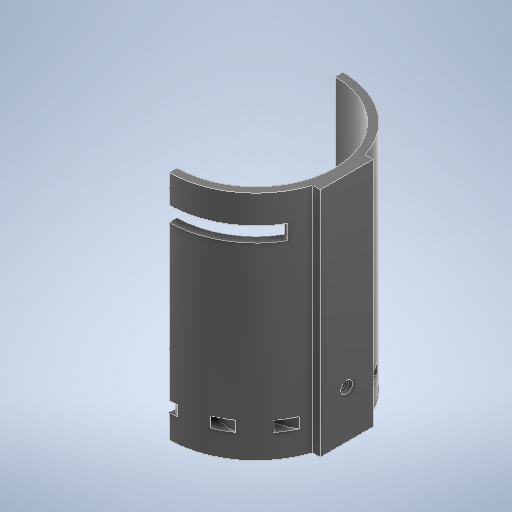
# Autodesk Inventor part: casing_cylindrical
Saved by Autodesk Inventor 2025 (Build 290162000, 162)
## iProperties
Created: 2026-08-03
Part Number: casing_cylindrical
Material: Ogólny
Document SubType Name: Modeling
Designer: zzapa
Density: 1 g/cm^3
Appearance: Gładki — czarny
Author: zzapa
Autodesk Inventor part; units mm, degrees
ref_plane "YZ Plane" through (0, 0, 0) normal (1, 0, 0) x (0, 1, 0)
ref_plane "XZ Plane" through (0, 0, 0) normal (0, 1, 0) x (-1, 0, 0)
sketch "Szkic1" plane through (0, 0, 0) normal (0, 0, 1) x (1, 0, 0)
  line L0 (-6.6, 0) -> (39.6, 0) projected
  line L1 (33, 80) -> (30, 80)
  line L2 (30, 80) -> (30, 0)
  line L3 (30, 0) -> (33, 0)
  line L4 (33, 0) -> (33, 80)
  line L5 (0, -29.6) -> (0, 121.6) projected
  line L6 (33, -8) -> (14, -8)
  line L7 (14, -8) -> (14, 0)
  line L8 (14, 0) -> (33, 0)
  line L9 (33, 0) -> (33, -8)
  line L10 (23, 6) -> (30, 6)
  line L11 (30, 6) -> (30, 0)
  line L12 (30, 0) -> (23, 0)
  line L13 (23, 0) -> (23, 6)
  point P0 (0, 0)
  point P1 (30, 0)
  point P2 (33, 0)
  point P3 (14, 0)
  point P4 (23, 0)
  dimension "d0" = 30
  dimension "d1" = 3
  dimension "d2" = 80
  dimension "d4" = 8
  dimension "d5" = 14
  dimension "d6" = 23
  dimension "d7" = 6
  constraints: 24 end point, 6 parallel, 5 collinear, 3 horizontal, 3 perpendicular
  measures "d0" distance from line of point (0, 0) L2
  measures "d1" distance of L1.start L1.end
  measures "d2" distance of L3.end L1.start
  measures "d4" distance of L6.end L7.end
  measures "d5" distance between parallel lines of L5 L7
  measures "d6" distance between parallel lines of L5 L13
  measures "d7" distance of L12.end L10.start
revolve "Obrót1" add sketch "Szkic1" angle 360 about axis through (0, -10, 0) along (0, 1, 0)
sketch "Szkic2" plane through (0, -8, 0) normal (0, -1, 0) x (1, 0, 0)
  circle A0 centre (0, 0) radius 33 projected
  line L0 (-34.4484, 10) -> (-31.4484, 10)
  line L1 (-31.4484, 10) -> (-31.4484, -10)
  line L2 (-31.4484, -10) -> (-34.4484, -10)
  line L3 (-34.4484, -10) -> (-34.4484, 10)
  line L4 (0, -46.2) -> (0, 46.2) projected
  line L5 (34.4484, 10) -> (31.4484, 10)
  line L6 (31.4484, 10) -> (31.4484, -10)
  line L7 (31.4484, -10) -> (34.4484, -10)
  line L8 (34.4484, -10) -> (34.4484, 10)
  line L9 (-49.8666, 0) -> (49.8666, 0) projected
  point P0 (-31.4484, 0)
  dimension "d10" = 20
  dimension "d11" = 3
  constraints: 16 end point, 4 symmetric about line, 2 parallel, 1 horizontal, 1 midpoint, 1 perpendicular, 1 point on line, 2 other
  measures "d10" distance of L2.end L0.start
  measures "d11" distance from line of L3 point (-31.448, 0)
extrude "Wyciągnięcie proste1" add sketch "Szkic2" against normal up to surface (88 mm away) contours L9 L6 A0 | L9 L8 L7 A0 | A0 L6 L9 | A0 L5 L8 L9 | L1 L9 A0 | A0 L9 L3 L0 | L2 L3 L9 A0 | A0 L9 L1
ref_plane "Płaszczyzna konstrukcyjna1" through (0, 36, 33) normal (0, 0, 1) x (1, 0, 0)
sketch "Szkic3" plane through (0, 36, 33) normal (0, 0, 1) x (1, 0, 0)
  line L0 (3.5, -35) -> (-3.5, -35)
  line L1 (-3.5, -35) -> (-3.5, -31)
  line L2 (-3.5, -31) -> (3.5, -31)
  line L3 (3.5, -31) -> (3.5, -35)
  line L4 (23, -36) -> (-23, -36) projected
  line L5 (23, -30) -> (-23, -30) projected
  line L6 (0, -30) -> (0, -36)
  line L7 (-3.5, -31) -> (3.5, -35)
  point P0 (0, -35)
  point P1 (0, -33)
  dimension "d17" = 4
  dimension "d18" = 7
  constraints: 12 end point, 4 midpoint, 2 parallel, 1 horizontal, 1 perpendicular
  measures "d17" distance of L2.end L0.start
  measures "d18" distance of L1.end L2.end
sketch "Szkic4" plane through (0, 6, 0) normal (0, 1, 0) x (1, 0, 0)
  arc A0 (-31.4484, -10) -> (31.4484, -10) centre (0, 0) ccw projected
  arc A1 (0, 0) -> (0, -33) centre (11.3027, -16.5) ccw
  dimension "d19" = 20
  constraints: 4 point on circle, 1 centre point, 1 coincident
  measures "d19" radius of A1
sweep "Przeciągnięcie1" cut profiles "Szkic3" path "Szkic4" path curves A1
pattern_circular "Szyk kołowy1" count 12 over 360 about axis through (0, -10, 0) along (0, 1, 0) of "Przeciągnięcie1" skipped copies 4 10
sketch "Szkic5" plane through (-34.4484, -8, 10) normal (0, -1, 0) x (1, 0, 0)
  line L0 (34.4484, -56.2) -> (34.4484, 36.2) projected
  point P0 (34.4484, -10)
  point P1 (34.4484, 9)
  point P2 (17.9939, -19.5)
  point P3 (50.9029, -19.5)
  dimension "d20" = 19
  dimension "d23" = 360
  constraints: 1 point on line, 4 other
  measures "d20" distance of point (34.448, -10) point (34.448, 9)
hole "Otwór1" at (0, -8, 19) at (-16.4545, -8, -9.5) at (16.4545, -8, -9.5) direction (0, 1, 0) diameter 2.9 end through all
sketch "Szkic6" plane through (-34.4484, -8, -10) normal (-1, 0, 0) x (0, 0, 1)
  line L0 (10, -17.6) -> (10, 105.6) projected
  line L1 (20, 0) -> (0, 0) projected
  point P0 (10, 8)
  point P1 (10, 18.1)
  dimension "d35" = 18.1
  constraints: 1 point on line
  measures "d35" distance from line of L1 point (10, 18.1)
hole "Otwór2" at (-34.4484, 10.1, 0) direction (1, 0, 0) diameter 2.6 depth 34.4484 counterbore diameter 4.5 counterbore depth 1.5
mirror "Odbij1" about plane through (0, 0, 0) normal (1, 0, 0) of "Otwór2"
chamfer "Faza1" distance 0.5 angle 45 3 edges at (0, -8, 20.45) (-16.4545, -8, -8.05) (16.4545, -8, -8.05)
sketch "Szkic7" plane through (0, 0, 0) normal (1, 0, 0) x (0, 1, 0)
  line L0 (-25.6, 0) -> (97.6, 0) projected
  line L1 (69.2446, 30) -> (63.5805, 30)
  line L2 (63.5805, 30) -> (63.5805, 33)
  line L3 (63.5805, 33) -> (69.2446, 33)
  line L4 (69.2446, 33) -> (69.2446, 30)
  line L5 (5, 26.5291) -> (5, 30.0369) projected
  line L6 (5, 30.0369) -> (1, 30.0369) projected
  line L7 (1, 30.0369) -> (1, 26.5291) projected
  line L8 (1, 26.5291) -> (5, 26.5291) projected
  line L9 (5, 13.1615) -> (5, 19.1794) projected
  line L10 (5, 19.1794) -> (1, 19.1794) projected
  line L11 (1, 19.1794) -> (1, 13.1615) projected
  line L12 (1, 13.1615) -> (5, 13.1615) projected
  line L13 (1, 13.6668) -> (1, 19.6267) projected
  line L14 (1, 19.6267) -> (5, 19.6267) projected
  line L15 (5, 19.6267) -> (5, 13.6668) projected
  line L16 (5, 13.6668) -> (1, 13.6668) projected
  line L17 (1, 26.8543) -> (1, 30.2618) projected
  line L18 (1, 30.2618) -> (5, 30.2618) projected
  line L19 (5, 30.2618) -> (5, 26.8543) projected
  line L20 (5, 26.8543) -> (1, 26.8543) projected
  line L21 (1, 32.8462) -> (1, 32.7882) projected
  line L22 (1, 32.7882) -> (5, 32.7882) projected
  line L23 (5, 32.7882) -> (5, 32.8462) projected
  line L24 (5, 32.8462) -> (1, 32.8462) projected
  line L25 (-8, 10) -> (80, 10) projected
  line L26 (80, 10) -> (80, 10) projected
  line L27 (80, 10) -> (-8, 10) projected
  line L28 (-8, 10) -> (-8, 10) projected
  line L29 (-8, 33) -> (80, 33) projected
  line L30 (80, 30) -> (6, 30) projected
  point P0 (0, 0)
  constraints: 8 end point, 2 collinear, 2 parallel, 1 horizontal, 1 perpendicular
revolve "Obrót2" cut sketch "Szkic7" angle 120 mid plane about axis through (0, -10, 0) along (0, 1, 0) contours L1 L2 L3 L4
equation "\"d0\" = casing_r_in"
equation "\"d1\" = casing_d"
equation "\"d2\" = casing_h"
equation "\"d4\" = casing_lock_h"
equation "\"d5\" = casing_lock_hole_r"
equation "\"d6\" = casing_stator_fix_r"
equation "\"d7\" = casing_stator_fix_h"
equation "\"d10\" = casing_sidebar_width"
equation "\"d11\" = casing_sidebar_length"
equation "\"d17\" = casing_vent_hole_length"
equation "\"d18\" = casing_vent_hole_width"
equation "\"d19\" = casing_vent_hole_arc"
equation "\"d20\" = casing_head_insert_r"
equation "\"d25\" = insert_m2_d"
equation "\"d35\" = casing_radial_stator_insert_pos"
equation "\"d36\" = insert_m2_pocket_d"
equation "\"d38\" = insert_m2_pocket_D"
equation "\"d39\" = insert_m2_pocket_nut_h"
equation "\"d32\" = insert_m2_corner"
equation "\"stator_out_d\" = 2.5"
equation "\"stator_h\" = 45"
equation "\"mag_size_x\" = 7"
equation "\"mag_size_y\" = 3"
equation "\"mag_corner_r\" = 0.4"
equation "\"magnet_ring_r\" = 27.5"
equation "\"magnet_ring_d\" = 3.3"
equation "\"magnet_ring_h\" = 36"
equation "\"magnet_ring_pocket_mag_size_x\" = 7.1"
equation "\"magnet_ring_pocket_mag_size_y\" = 3.1"
equation "\"magnet_ring_pocket_mag_size_z\" = 10.3"
equation "\"magnet_ring_pocket_radial_cut\" = 1.4"
equation "\"casing_h\" = 80"
equation "\"casing_d\" = 3"
equation "\"casing_r_in\" = 30"
equation "\"rotor_core_r\" = 15"
equation "\"coil_groove_ang\" = 18"
equation "\"rotor_out_r\" = 23"
equation "\"rotor_coil_groove_in_r\" = 17"
equation "\"rotor_coil_groove_ang\" = 18deg"
equation "\"rotor_coil_groove_in_correction_r\" = 18"
equation "\"rotor_plastic_h\" = 32"
equation "\"rotor_teeth_d\" = 1.5"
equation "\"shaft_d\" = 8"
equation "\"insert25m_d\" = 2.9"
equation "\"insert25m_corner\" = 0.5"
equation "\"insert25m_h\" = 7"
equation "\"rotor_plastic_insert_r\" = 37"
equation "\"shaft_lock_1_d\" = 8"
equation "\"shaf_lock_1_D\" = 32"
equation "\"shaft_lock_1_D\" = 44"
equation "\"shaft_lock_1_h1\" = 3.5"
equation "\"shaft_lock_1_insert_part_h\" = 8"
equation "\"shaft_lock_1_corner\" = 2"
equation "\"shaft_lock_1_insert_part_a\" = 18"
equation "\"shaft_lock_2_h1\" = 3.5"
equation "\"shaft_lock_2_d\" = 8"
equation "\"shaft_lock_2_insert_part_a\" = 18"
equation "\"shaft_lock_2_D\" = 44"
equation "\"shaft_lock_2_corner\" = 2"
equation "\"shaft_lock_2_insert_part_h\" = 7"
equation "\"shaft_lock_2_rotor_insert_grove_d_in\" = 36"
equation "\"shaft_lock_2_rotor_insert_grove_width_out\" = 5.5"
equation "\"shaft_lock_2_rotor_insert_grove_width_in\" = 7.6"
equation "\"shaft_lock_2_rotor_insert_r\" = 37"
equation "\"shaft_lock_2_rotor_insert_screw_d\" = 2.6"
equation "\"insert25m_pocket_d\" = 2.6"
equation "\"insert25m_pocket_D\" = 4.5"
equation "\"insert25m_pocket_nut_h\" = 1.5"
equation "\"insert_m2_pocket_d\" = 2.6"
equation "\"insert_m2_h\" = 7"
equation "\"insert_m2_d\" = 2.9"
equation "\"insert_m2_corner\" = 0.5"
equation "\"insert_m2_pocket_D\" = 4.5"
equation "\"insert_m2_pocket_nut_h\" = 1.5"
equation "\"shaft_lock_1_insert_part_corner\" = 6"
equation "\"shaft_lock_1_insert_part_pos\" = 4"
equation "\"shaft_lock_1_rotor_insert_grove_width_in\" = 7.6"
equation "\"shaft_lock_1_rotor_insert_r\" = 37"
equation "\"shaft_lock_1_rotor_insert_grove_d_in\" = 36"
equation "\"shaft_lock_1_rotor_insert_grove_width_out\" = 5.5"
equation "\"shaft_lock_1_shaft_insert_axial_cut_out_width\" = 12"
equation "\"shaft_lock_1_shaft_insert_axial_cut_in_width\" = 5.4"
equation "\"shaft_lock_1_shaft_insert_corner\" = 2"
equation "\"shaft_lock_1_shaft_insert_corner_finish\" = 0.5"
equation "\"shaft_lock_1_shaft_insert_pos\" = 2.5"
equation "\"shaft_lock_2_shaft_insert_corner\" = 2"
equation "\"shaft_lock_2_shaft_insert_pos\" = 2.5"
equation "\"shaft_lock_2_shaft_insert_axial_cut_in_width\" = 5.4"
equation "\"shaft_lock_2_shaft_insert_axial_cut_out_width\" = 12"
equation "\"shaft_lock_2_shaft_insert_corner_finish\" = 0.5"
equation "\"commutator_plate_D\" = 22"
equation "\"commutator_plastic_d\" = 1"
equation "\"commutator_plastic_h\" = 15"
equation "\"commutator_plate_ang\" = 55deg"
equation "\"commutator_plate_d\" = 1"
equation "\"commutator_plate_h\" = 15"
equation "\"commutator_plastic_shaft_d\" = 8"
equation "\"commutator_plastic_insert_cut_deepness\" = 1"
equation "\"commutator_plastic_insert_cut_length\" = 6"
equation "\"commutator_plastic_insert_pos\" = 3"
equation "\"commutator_plate_insert_pos\" = 3"
equation "\"casing_lock_hole_r\" = 14"
equation "\"casing_lock_h\" = 8"
equation "\"casing_stator_fix_r\" = 23"
equation "\"casing_stator_fix_h\" = 6"
equation "\"magnet_ring_insert_part_lengthen\" = 8"
equation "\"casing_sidebar_width\" = 20"
equation "\"casing_sidebar_length\" = 3"
equation "\"casing_vent_hole_length\" = 4"
equation "\"casing_vent_hole_width\" = 7"
equation "\"casing_vent_hole_arc\" = 20"
equation "\"sleeve_cup_r\" = 22"
equation "\"sleeve_cup_h\" = 3"
equation "\"sleeve_d\" = 3"
equation "\"sleeve_in_r\" = 11"
equation "\"casing_head_insert_r\" = 19"
equation "\"sleeve_head_insert_r\" = 19"
equation "\"magnet_ring_insert_part_radius_cut\" = 0.17"
equation "\"magnet_ring_insert_part_axial_flat_cut\" = 0.17"
equation "\"magnet_ring_insert_pos\" = 4"
equation "\"casing_radial_stator_insert_pos\" = 18.1"
equation "\"stator_radial_screw_d\" = 4"
equation "\"stator_radial_screw_pos\" = 4"
equation "\"rotor_sleeve_out_D\" = 10.5"
equation "\"rotor_sleeve_in_D\" = 8"
equation "\"rotor_sleeve_h\" = 32"
equation "\"carbon_brush_batt_d\" = 5"
